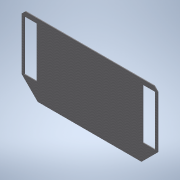
# Autodesk Inventor part: plancah base
Saved by Autodesk Inventor 2022.1 (Build 261234000, 234)
## iProperties
Created: 2021-09-11
Part Number: plancah base
Material: Steel, Mild, Welded
Document SubType Name: Modeling
Designer: Andres
Density: 7.85 g/cm^3
Appearance: Weld - Steel Mild
Author: Andres
Autodesk Inventor part; units mm, degrees
ref_plane "YZ Plane" through (0, 0, 0) normal (1, 0, 0) x (0, 1, 0)
ref_plane "XZ Plane" through (0, 0, 0) normal (0, 1, 0) x (-1, 0, 0)
ref_plane "XY Plane" through (0, 0, 0) normal (0, 0, 1) x (1, 0, 0)
sketch "Sketch1" plane through (0, 0, 0) normal (0, 0, 1) x (1, 0, 0)
  line L0 (-318, 277.5147) -> (-330, 282.4853) projected
  line L1 (-330, 282.4853) -> (-330, -52.4853) projected
  line L2 (-330, -52.4853) -> (-318, -47.5147) projected
  line L3 (-318, 277.5147) -> (-318, -47.5147) projected
  line L4 (-318, -47.5147) -> (-330, -52.4853) projected
  line L5 (-330, -52.4853) -> (-226.4853, -156) projected
  line L6 (-226.4853, -156) -> (-221.5147, -144) projected
  line L7 (-318, -47.5147) -> (-221.5147, -144) projected
  line L8 (-330, 282.4853) -> (-318, 277.5147) projected
  line L9 (-301.5147, 294) -> (-318, 277.5147) projected
  line L10 (-301.5147, 294) -> (-306.4853, 306) projected
  line L11 (-306.4853, 306) -> (-330, 282.4853) projected
  line L12 (-306.4853, 306) -> (-301.5147, 294) projected
  line L13 (513.5147, 294) -> (-301.5147, 294) projected
  line L14 (513.5147, 294) -> (518.4853, 306) projected
  line L15 (518.4853, 306) -> (-306.4853, 306) projected
  line L16 (542, 282.4853) -> (518.4853, 306) projected
  line L17 (530, 277.5147) -> (542, 282.4853) projected
  line L18 (542, 282.4853) -> (518.4853, 306) projected
  line L19 (518.4853, 306) -> (513.5147, 294) projected
  line L20 (530, 277.5147) -> (513.5147, 294) projected
  line L21 (530, -47.5147) -> (542, -52.4853) projected
  line L22 (542, -52.4853) -> (542, 282.4853) projected
  line L23 (542, 282.4853) -> (530, 277.5147) projected
  line L24 (530, -47.5147) -> (530, 277.5147) projected
  line L25 (433.5147, -144) -> (438.4853, -156) projected
  line L26 (438.4853, -156) -> (542, -52.4853) projected
  line L27 (542, -52.4853) -> (530, -47.5147) projected
  line L28 (433.5147, -144) -> (530, -47.5147) projected
  line L29 (-221.5147, -144) -> (-226.4853, -156) projected
  line L30 (-226.4853, -156) -> (438.4853, -156) projected
  line L31 (438.4853, -156) -> (433.5147, -144) projected
  line L32 (-221.5147, -144) -> (433.5147, -144) projected
  line L33 (445.8717, 275.4134) -> (485.8717, 275.4134)
  line L34 (485.8717, 275.4134) -> (485.8717, 125.4134)
  line L35 (445.8717, 125.4134) -> (445.8717, 275.4134)
  line L36 (485.8717, 125.4134) -> (445.8717, 125.4134)
  point P0 (0, 0)
  constraints: 8 end point, 2 horizontal, 2 vertical, 4 other
extrude "Extrusion1" add sketch "Sketch1" along normal blind 5 contours L3 L2 L1 L0 | L9 L13 L20 L24 L28 L32 L7 L3 | L0 L11 L10 L9 | L7 L6 L5 L2 | L10 L15 L14 L13 | L32 L25 L30 L6 | L14 L16 L17 L20 | L28 L21 L26 L25 | L17 L22 L21 L24 | L33 L34 L36 L35
sketch "Boceto4" plane through (0, 0, 5) normal (0, 0, 1) x (1, 0, 0)
  line L0 (-330, 282.4853) -> (-330, -52.4853) projected
  line L1 (-208, -144) -> (-208, 294) projected
  line L2 (-314, 275.8579) -> (-314, -45.8579) projected
  line L3 (-314, -45.8579) -> (-234, -45.8579)
  line L4 (-314, 275.8579) -> (-234, 275.8579)
  line L5 (-234, -45.8579) -> (-234, 275.8579)
  line L6 (-314, -45.8579) -> (-314, 275.8579)
  line L7 (526, -45.8579) -> (526, 275.8579) projected
  line L8 (426, 290) -> (426, -140) projected
  line L9 (446, -45.8579) -> (446, 275.8579)
  line L10 (446, -45.8579) -> (526, -45.8579)
  line L11 (446, 275.8579) -> (526, 275.8579)
  point P0 (0, 0)
  point P1 (426, 4.1421)
  point P2 (426, 275.8579)
  dimension "d8" = 80
  dimension "d10" = 80
  constraints: 14 end point, 3 parallel, 2 perpendicular, 2 point on line
  measures "d8" distance between parallel lines of L5 L2
  measures "d10" distance between parallel lines of L7 L9
extrude "Extrusión4" cut sketch "Boceto4" against normal blind 20
body "Solid1"
